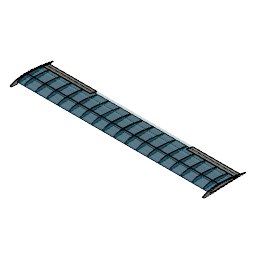
wing (Autodesk Fusion 360 design; units mm, degrees)
part number: 2026-03-18-19-06-06-757
Autodesk Fusion 360 part; units mm, degrees
(part 1 of 3)
ref_plane "WorkPlane1" through (0, 0, 0) normal (0, 0, 1) x (1, 0, 0)
sketch "Sketch2" plane through (0, 0, 0) normal (1, 0, 0) x (0, 1, 0)
  spline S0 degree 5 poles (61.12, 19.8844) (61.603, 19.9031) (62.5903, 19.9386) (64.1373, 19.9858) (66.3336, 20.0363) (69.2771, 20.0768) (72.3733, 20.092) (75.5651, 20.0792) (78.7922, 20.0358) (82.0002, 19.9602) (85.1491, 19.852) (88.221, 19.7125) (91.2143, 19.5444) (94.1405, 19.3507) (97.0192, 19.1349) (99.8745, 18.9002) (102.7305, 18.6492) (105.6069, 18.383) (108.5159, 18.1017) (111.4639, 17.8039) (114.4514, 17.4884) (117.4739, 17.1533) (120.5226, 16.7977) (123.585, 16.421) (126.6452, 16.0244) (129.6857, 15.6102) (132.6897, 15.1815) (135.6441, 14.7413) (138.5414, 14.2923) (141.3828, 13.8358) (144.1802, 13.3716) (146.96, 12.8967) (149.7596, 12.4062) (152.6192, 11.8943) (155.5748, 11.3555) (158.65, 10.7855) (161.8488, 10.1828) (165.1491, 9.5491) (168.4917, 8.8914) (171.7902, 8.2207) (174.9494, 7.5502) (177.8817, 6.8932) (180.5234, 6.2618) (182.8532, 5.6644) (184.9056, 5.1048) (186.7958, 4.5791) (188.6853, 4.0776) (190.7296, 3.5872) (193.0295, 3.0932) (195.585, 2.582) (198.2365, 2.0427) (200.7124, 1.4729) (202.699, 0.8841) (203.9033, 0.3094) (204.1194, -0.195) (203.2912, -0.5318) (201.5529, -0.6648) (199.1776, -0.6277) (196.496, -0.4891) (193.8227, -0.3307) (191.3831, -0.2214) (189.2303, -0.1908) (187.2848, -0.2357) (185.3935, -0.3335) (183.381, -0.4524) (181.1051, -0.5633) (178.5092, -0.6507) (175.6031, -0.7098) (172.4448, -0.7441) (169.123, -0.7621) (165.7378, -0.7755) (162.3835, -0.7955) (159.1292, -0.8308) (156.004, -0.8848) (153.0074, -0.9575) (150.117, -1.0461) (147.2962, -1.146) (144.5027, -1.2521) (141.6962, -1.3598) (138.8471, -1.4658) (135.9416, -1.5694) (132.9775, -1.6708) (129.9619, -1.7717) (126.9085, -1.8739) (123.8347, -1.9795) (120.7588, -2.0898) (117.6975, -2.2052) (114.6637, -2.3247) (111.6664, -2.4469) (108.7102, -2.5697) (105.7944, -2.6913) (102.9129, -2.8103) (100.0533, -2.9259) (97.1963, -3.039) (94.3176, -3.1511) (91.3932, -3.2647) (88.403, -3.3821) (85.3351, -3.5056) (82.1901, -3.6364) (78.985, -3.7745) (75.7583, -3.9183) (72.564, -4.0644) (69.462, -4.2092) (66.5097, -4.3487) (63.7533, -4.4796) (61.2187, -4.5998) (58.9035, -4.7092) (56.7672, -4.8101) (54.7458, -4.9063) (52.7684, -5.0022) (50.7726, -5.101) (48.7209, -5.2041) (46.615, -5.3099) (44.4793, -5.4149) (42.347, -5.5148) (40.2457, -5.6055) (38.181, -5.6845) (36.1282, -5.7511) (34.0511, -5.8058) (31.9176, -5.8493) (29.714, -5.8817) (27.4654, -5.9014) (25.2368, -5.9054) (23.1072, -5.8903) (21.1491, -5.8545) (19.4072, -5.799) (17.8722, -5.7297) (16.4825, -5.6547) (15.1531, -5.5769) (13.7964, -5.4879) (12.345, -5.3623) (10.7731, -5.1743) (9.1101, -4.9106) (7.4743, -4.59) (6.019, -4.2496) (4.8464, -3.9155) (3.9079, -3.575) (2.9736, -3.1567) (1.8623, -2.5675) (0.722, -1.7188) (-0.0619, -0.564) (-0.1465, 0.8714) (0.4773, 2.4376) (1.5165, 3.9094) (2.6176, 5.0911) (3.5469, 5.9078) (4.3846, 6.494) (5.3418, 7.0607) (6.5667, 7.749) (8.0285, 8.5465) (9.6168, 9.3729) (11.1943, 10.128) (12.6796, 10.7659) (14.0587, 11.2993) (15.3629, 11.7682) (16.6574, 12.2197) (18.0246, 12.6838) (19.543, 13.177) (21.2669, 13.7028) (23.2007, 14.2542) (25.2995, 14.8155) (27.4942, 15.3676) (29.7097, 15.8913) (31.8851, 16.3717) (33.9968, 16.8029) (36.0579, 17.1875) (38.0987, 17.5329) (40.1536, 17.8487) (42.246, 18.1437) (44.3706, 18.4219) (46.5002, 18.6835) (48.602, 18.9264) (50.6512, 19.1472) (52.6451, 19.3434) (54.619, 19.5144) (56.6343, 19.6612) (58.3363, 19.7608) (59.6922, 19.8261) (60.637, 19.8656) (61.12, 19.8844) knots 0 0 0 0 0 0 0.00571429 0.01142857 0.01714286 0.02285714 0.02857143 0.03428571 0.04 0.04571429 0.05142857 0.05714286 0.06285714 0.06857143 0.07428571 0.08 0.08571429 0.09142857 0.09714286 0.10285714 0.10857143 0.11428571 0.12 0.12571429 0.13142857 0.13714286 0.14285714 0.14857143 0.15428571 0.16 0.16571429 0.17142857 0.17714286 0.18285714 0.18857143 0.19428571 0.2 0.20571429 0.21142857 0.21714286 0.22285714 0.22857143 0.23428571 0.24 0.24571429 0.25142857 0.25714286 0.26285714 0.26857143 0.27428571 0.28 0.28571429 0.29142857 0.29714286 0.30285714 0.30857143 0.31428571 0.32 0.32571429 0.33142857 0.33714286 0.34285714 0.34857143 0.35428571 0.36 0.36571429 0.37142857 0.37714286 0.38285714 0.38857143 0.39428571 0.4 0.40571429 0.41142857 0.41714286 0.42285714 0.42857143 0.43428571 0.44 0.44571429 0.45142857 0.45714286 0.46285714 0.46857143 0.47428571 0.48 0.48571429 0.49142857 0.49714286 0.50285714 0.50857143 0.51428571 0.52 0.52571429 0.53142857 0.53714286 0.54285714 0.54857143 0.55428571 0.56 0.56571429 0.57142857 0.57714286 0.58285714 0.58857143 0.59428571 0.6 0.60571429 0.61142857 0.61714286 0.62285714 0.62857143 0.63428571 0.64 0.64571429 0.65142857 0.65714286 0.66285714 0.66857143 0.67428571 0.68 0.68571429 0.69142857 0.69714286 0.70285714 0.70857143 0.71428571 0.72 0.72571429 0.73142857 0.73714286 0.74285714 0.74857143 0.75428571 0.76 0.76571429 0.77142857 0.77714286 0.78285714 0.78857143 0.79428571 0.8 0.80571429 0.81142857 0.81714286 0.82285714 0.82857143 0.83428571 0.84 0.84571429 0.85142857 0.85714286 0.86285714 0.86857143 0.87428571 0.88 0.88571429 0.89142857 0.89714286 0.90285714 0.90857143 0.91428571 0.92 0.92571429 0.93142857 0.93714286 0.94285714 0.94857143 0.95428571 0.96 0.96571429 0.97142857 0.97714286 0.98285714 0.98857143 0.99428571 1 1 1 1 1 1
  line L0 (0, 0) -> (203.9051, -0.0198) construction
  point P0 (203.7334, 0.2649)
  point P1 (193.5467, 2.9949)
  point P2 (183.3601, 5.5212)
  point P3 (162.9867, 9.9626)
  point P4 (142.6134, 13.6298)
  point P5 (122.24, 16.5839)
  point P6 (101.8667, 18.7231)
  point P7 (81.4934, 19.9659)
  point P8 (61.12, 19.8844)
  point P9 (50.9334, 19.1713)
  point P10 (40.7467, 17.9285)
  point P11 (30.56, 16.0746)
  point P12 (20.3733, 13.426)
  point P13 (15.28, 11.735)
  point P14 (10.1867, 9.6366)
  point P15 (5.0933, 6.9066)
  point P16 (2.5467, 4.9711)
  point P17 (2.5467, -2.9134)
  point P18 (5.0933, -3.9728)
  point P19 (10.1867, -5.073)
  point P20 (15.28, -5.5823)
  point P21 (20.3733, -5.8268)
  point P22 (30.56, -5.8675)
  point P23 (40.7467, -5.5823)
  point P24 (50.9334, -5.0933)
  point P25 (61.12, -4.6044)
  point P26 (81.4934, -3.6672)
  point P27 (101.8667, -2.8523)
  point P28 (122.24, -2.0373)
  point P29 (142.6134, -1.3243)
  point P30 (162.9867, -0.7946)
  point P31 (183.3601, -0.4482)
  point P32 (193.5467, -0.326)
  point P33 (203.7334, -0.2649)
  point P34 (81.4934, 19.9659)
  point P35 (101.8667, 18.7231)
  point P36 (122.24, 16.5839)
  point P37 (142.6134, 13.6298)
  point P38 (162.9867, 9.9626)
  point P39 (183.3601, 5.5212)
  point P40 (193.5467, 2.9949)
  point P41 (203.7334, 0.2649)
  point P42 (203.7334, -0.2649)
  point P43 (193.5467, -0.326)
  point P44 (183.3601, -0.4482)
  point P45 (162.9867, -0.7946)
  point P46 (142.6134, -1.3243)
  point P47 (122.24, -2.0373)
  point P48 (101.8667, -2.8523)
  point P49 (81.4934, -3.6672)
  point P50 (61.12, -4.6044)
  point P51 (50.9334, -5.0933)
  point P52 (40.7467, -5.5823)
  point P53 (30.56, -5.8675)
  point P54 (20.3733, -5.8268)
  point P55 (15.28, -5.5823)
  point P56 (10.1867, -5.073)
  point P57 (5.0933, -3.9728)
  point P58 (2.5467, -2.9134)
  point P59 (2.5467, 4.9711)
  point P60 (5.0933, 6.9066)
  point P61 (10.1867, 9.6366)
  point P62 (15.28, 11.735)
  point P63 (20.3733, 13.426)
  point P64 (30.56, 16.0746)
  point P65 (40.7467, 17.9285)
  point P66 (50.9334, 19.1713)
  constraint coincident P8 S0.start
  constraint coincident P34 P7
  constraint coincident P35 P6
  constraint coincident P36 P5
  constraint coincident P37 P4
  constraint coincident P38 P3
  constraint coincident P39 P2
  constraint coincident P40 P1
  constraint coincident P41 P0
  constraint coincident P42 P33
  constraint coincident P43 P32
  constraint coincident P44 P31
  constraint coincident P45 P30
  constraint coincident P46 P29
  constraint coincident P47 P28
  constraint coincident P48 P27
  constraint coincident P49 P26
  constraint coincident P50 P25
  constraint coincident P51 P24
  constraint coincident P52 P23
  constraint coincident P53 P22
  constraint coincident P54 P21
  constraint coincident P55 P20
  constraint coincident P56 P19
  constraint coincident P57 P18
  constraint coincident P58 P17
  constraint coincident L0.start origin
  constraint coincident P59 P16
  constraint coincident P60 P15
  constraint coincident P61 P14
  constraint coincident P62 P13
  constraint coincident P63 P12
  constraint coincident P64 P11
  constraint coincident P65 P10
  constraint coincident P66 P9
  constraint coincident S0 L0.end
sketch "Sketch3" plane through (0, 0, 0) normal (0, 0, 1) x (1, 0, 0)
  line L0 (0, 0) -> (0, 200)
  line L1 (299, 155) -> (299, 200)
  line L2 (301, 200) -> (301, 155)
  line L3 (301, 155) -> (599, 155)
  line L4 (599, 155) -> (599, 200)
  line L5 (599, 200) -> (301, 200)
  line L6 (-599, 155) -> (-599, 200)
  line L7 (-301, 200) -> (-301, 155)
  line L8 (-599, 200) -> (-301, 200)
  line L9 (-299, 155) -> (-299, 200)
  line L10 (-301, 155) -> (-599, 155)
  dimension "d9" = 298
  dimension "d10" = 301
  constraint coincident L0.start origin
  constraint vertical L0
  constraint horizontal L0.end L1.end
  constraint perpendicular L2 L3
  constraint perpendicular L3 L4
  constraint perpendicular L2 L5
  constraint symmetric L0 L1.start L9.start
  constraint symmetric L0 L1.end L9.end
  constraint symmetric L0 L2.start L7.start
  constraint symmetric L0 L2.end L7.end
  constraint symmetric L0 L3.end L6.start
  constraint symmetric L0 L4.end L6.end
  measures "d9" distance of L2 L4
  measures "d10" distance of L0 L2
ref_plane "WorkPlane3" through (600, 0, 0) normal (1, 0, 0) x (0, 1, 0)
sketch "Sketch4" plane through (600, 0, 0) normal (1, 0, 0) x (0, 1, 0)
  spline S0 degree 5 poles (61.12, 19.8844) (60.637, 19.8656) (59.6922, 19.8261) (58.3363, 19.7608) (56.6343, 19.6612) (54.619, 19.5144) (52.6451, 19.3434) (50.6512, 19.1472) (48.602, 18.9264) (46.5002, 18.6835) (44.3706, 18.4219) (42.246, 18.1437) (40.1536, 17.8487) (38.0987, 17.5329) (36.0579, 17.1875) (33.9968, 16.8029) (31.8851, 16.3717) (29.7097, 15.8913) (27.4942, 15.3676) (25.2995, 14.8155) (23.2007, 14.2542) (21.2669, 13.7028) (19.543, 13.177) (18.0246, 12.6838) (16.6574, 12.2197) (15.3629, 11.7682) (14.0587, 11.2993) (12.6796, 10.7659) (11.1943, 10.128) (9.6168, 9.3729) (8.0285, 8.5465) (6.5667, 7.749) (5.3418, 7.0607) (4.3846, 6.494) (3.5469, 5.9078) (2.6176, 5.0911) (1.5165, 3.9094) (0.4773, 2.4376) (-0.1465, 0.8714) (-0.0619, -0.564) (0.722, -1.7188) (1.8623, -2.5675) (2.9736, -3.1567) (3.9079, -3.575) (4.8464, -3.9155) (6.019, -4.2496) (7.4743, -4.59) (9.1101, -4.9106) (10.7731, -5.1743) (12.345, -5.3623) (13.7964, -5.4879) (15.1531, -5.5769) (16.4825, -5.6547) (17.8722, -5.7297) (19.4072, -5.799) (21.1491, -5.8545) (23.1072, -5.8903) (25.2368, -5.9054) (27.4654, -5.9014) (29.714, -5.8817) (31.9176, -5.8493) (34.0511, -5.8058) (36.1282, -5.7511) (38.181, -5.6845) (40.2457, -5.6055) (42.347, -5.5148) (44.4793, -5.4149) (46.615, -5.3099) (48.7209, -5.2041) (50.7726, -5.101) (52.7684, -5.0022) (54.7458, -4.9063) (56.7672, -4.8101) (58.9035, -4.7092) (61.2187, -4.5998) (63.7533, -4.4796) (66.5097, -4.3487) (69.462, -4.2092) (72.564, -4.0644) (75.7583, -3.9183) (78.985, -3.7745) (82.1901, -3.6364) (85.3351, -3.5056) (88.403, -3.3821) (91.3932, -3.2647) (94.3176, -3.1511) (97.1963, -3.039) (100.0533, -2.9259) (102.9129, -2.8103) (105.7944, -2.6913) (108.7102, -2.5697) (111.6664, -2.4469) (114.6637, -2.3247) (117.6975, -2.2052) (120.7588, -2.0898) (123.8347, -1.9795) (126.9085, -1.8739) (129.9619, -1.7717) (132.9775, -1.6708) (135.9416, -1.5694) (138.8471, -1.4658) (141.6962, -1.3598) (144.5027, -1.2521) (147.2962, -1.146) (150.117, -1.0461) (153.0074, -0.9575) (156.004, -0.8848) (159.1292, -0.8308) (162.3835, -0.7955) (165.7378, -0.7755) (169.123, -0.7621) (172.4448, -0.7441) (175.6031, -0.7098) (178.5092, -0.6507) (181.1051, -0.5633) (183.381, -0.4524) (185.3935, -0.3335) (187.2848, -0.2357) (189.2303, -0.1908) (191.3831, -0.2214) (193.8227, -0.3307) (196.496, -0.4891) (199.1776, -0.6277) (201.5529, -0.6648) (203.2912, -0.5318) (204.1194, -0.195) (203.9033, 0.3094) (202.699, 0.8841) (200.7124, 1.4729) (198.2365, 2.0427) (195.585, 2.582) (193.0295, 3.0932) (190.7296, 3.5872) (188.6853, 4.0776) (186.7958, 4.5791) (184.9056, 5.1048) (182.8532, 5.6644) (180.5234, 6.2618) (177.8817, 6.8932) (174.9494, 7.5502) (171.7902, 8.2207) (168.4917, 8.8914) (165.1491, 9.5491) (161.8488, 10.1828) (158.65, 10.7855) (155.5748, 11.3555) (152.6192, 11.8943) (149.7596, 12.4062) (146.96, 12.8967) (144.1802, 13.3716) (141.3828, 13.8358) (138.5414, 14.2923) (135.6441, 14.7413) (132.6897, 15.1815) (129.6857, 15.6102) (126.6452, 16.0244) (123.585, 16.421) (120.5226, 16.7977) (117.4739, 17.1533) (114.4514, 17.4884) (111.4639, 17.8039) (108.5159, 18.1017) (105.6069, 18.383) (102.7305, 18.6492) (99.8745, 18.9002) (97.0192, 19.1349) (94.1405, 19.3507) (91.2143, 19.5444) (88.221, 19.7125) (85.1491, 19.852) (82.0002, 19.9602) (78.7922, 20.0358) (75.5651, 20.0792) (72.3733, 20.092) (69.2771, 20.0768) (66.3336, 20.0363) (64.1373, 19.9858) (62.5903, 19.9386) (61.603, 19.9031) (61.12, 19.8844) knots -1 -1 -1 -1 -1 -1 -0.99428571 -0.98857143 -0.98285714 -0.97714286 -0.97142857 -0.96571429 -0.96 -0.95428571 -0.94857143 -0.94285714 -0.93714286 -0.93142857 -0.92571429 -0.92 -0.91428571 -0.90857143 -0.90285714 -0.89714286 -0.89142857 -0.88571429 -0.88 -0.87428571 -0.86857143 -0.86285714 -0.85714286 -0.85142857 -0.84571429 -0.84 -0.83428571 -0.82857143 -0.82285714 -0.81714286 -0.81142857 -0.80571429 -0.8 -0.79428571 -0.78857143 -0.78285714 -0.77714286 -0.77142857 -0.76571429 -0.76 -0.75428571 -0.74857143 -0.74285714 -0.73714286 -0.73142857 -0.72571429 -0.72 -0.71428571 -0.70857143 -0.70285714 -0.69714286 -0.69142857 -0.68571429 -0.68 -0.67428571 -0.66857143 -0.66285714 -0.65714286 -0.65142857 -0.64571429 -0.64 -0.63428571 -0.62857143 -0.62285714 -0.61714286 -0.61142857 -0.60571429 -0.6 -0.59428571 -0.58857143 -0.58285714 -0.57714286 -0.57142857 -0.56571429 -0.56 -0.55428571 -0.54857143 -0.54285714 -0.53714286 -0.53142857 -0.52571429 -0.52 -0.51428571 -0.50857143 -0.50285714 -0.49714286 -0.49142857 -0.48571429 -0.48 -0.47428571 -0.46857143 -0.46285714 -0.45714286 -0.45142857 -0.44571429 -0.44 -0.43428571 -0.42857143 -0.42285714 -0.41714286 -0.41142857 -0.40571429 -0.4 -0.39428571 -0.38857143 -0.38285714 -0.37714286 -0.37142857 -0.36571429 -0.36 -0.35428571 -0.34857143 -0.34285714 -0.33714286 -0.33142857 -0.32571429 -0.32 -0.31428571 -0.30857143 -0.30285714 -0.29714286 -0.29142857 -0.28571429 -0.28 -0.27428571 -0.26857143 -0.26285714 -0.25714286 -0.25142857 -0.24571429 -0.24 -0.23428571 -0.22857143 -0.22285714 -0.21714286 -0.21142857 -0.20571429 -0.2 -0.19428571 -0.18857143 -0.18285714 -0.17714286 -0.17142857 -0.16571429 -0.16 -0.15428571 -0.14857143 -0.14285714 -0.13714286 -0.13142857 -0.12571429 -0.12 -0.11428571 -0.10857143 -0.10285714 -0.09714286 -0.09142857 -0.08571429 -0.08 -0.07428571 -0.06857143 -0.06285714 -0.05714286 -0.05142857 -0.04571429 -0.04 -0.03428571 -0.02857143 -0.02285714 -0.01714286 -0.01142857 -0.00571429 0 0 0 0 0 0
  spline S1 degree 3 poles (61.2364, 16.8866) (57.6324, 16.7467) (54.837, 16.5421) (51.8513, 16.2482) (49.2932, 15.9964) (46.5535, 15.6792) (43.8366, 15.324) (41.401, 15.0055) (39.0596, 14.6628) (36.7294, 14.2509) (34.6015, 13.8747) (32.4156, 13.4278) (30.1291, 12.901) (27.6916, 12.3395) (25.1848, 11.6956) (23.0631, 11.091) (21.2216, 10.5662) (19.7064, 10.0816) (18.3739, 9.632) (16.6918, 9.0644) (15.2258, 8.5644) (13.5524, 7.8653) (12.4462, 7.4031) (11.2189, 6.8194) (9.9999, 6.1844) (8.9215, 5.6226) (7.8857, 5.0512) (7.1019, 4.6035) (6.4838, 4.2504) (6.0525, 3.9896) (5.6921, 3.7303) (5.3517, 3.4854) (5.0032, 3.1949) (4.5699, 2.7504) (4.1116, 2.2804) (3.595, 1.6449) (3.2914, 1.117) (3.1087, 0.7992) (3.0156, 0.5398) (2.9897, 0.42) knots -1 -1 -1 -1 -0.97404 -0.97404 -0.97404 -0.951798 -0.951798 -0.951798 -0.931858 -0.931858 -0.931858 -0.913649 -0.913649 -0.913649 -0.894237 -0.894237 -0.894237 -0.877389 -0.877389 -0.877389 -0.856122 -0.856122 -0.856122 -0.842064 -0.842064 -0.842064 -0.829628 -0.829628 -0.829628 -0.819821 -0.819821 -0.819821 -0.810556 -0.810556 -0.810556 -0.800757 -0.800757 -0.800757 -0.79486 -0.79486 -0.79486 -0.79486
  spline S2 degree 3 poles (2.9897, 0.42) (3.0543, 0.3464) (3.1943, 0.219) (3.3872, 0.0837) (3.7574, -0.176) (4.273, -0.4422) (4.7124, -0.6375) (5.2684, -0.8846) (5.7621, -1.0583) (6.571, -1.2759) (7.6681, -1.5709) (9.285, -1.9057) (10.7983, -2.1313) (12.3486, -2.3624) (13.7433, -2.4772) (15.0921, -2.5644) (16.7453, -2.6714) (18.3654, -2.7647) (20.5139, -2.8297) (22.493, -2.8895) (24.9582, -2.9109) (27.506, -2.8972) (29.7799, -2.8851) (32.0483, -2.8498) (34.1902, -2.7985) (36.8126, -2.7357) (39.3288, -2.6442) (41.9726, -2.5266) (44.569, -2.411) (47.2437, -2.2742) (49.7746, -2.1475) (52.1544, -2.0283) (54.3796, -1.9201) (56.8136, -1.8047) (59.0608, -1.6981) (61.5509, -1.5807) (64.4566, -1.4428) (69.9758, -1.181) (76.92, -0.8547) (83.3434, -0.5864) (87.9529, -0.3939) (92.2873, -0.2286) (96.4895, -0.064) (101.2103, 0.121) (105.8624, 0.3155) (110.7376, 0.5168) (116.1156, 0.7389) (121.7528, 0.9526) (127.3, 1.1404) (131.5605, 1.2846) (135.7191, 1.4217) (139.6944, 1.5684) (145.3748, 1.778) (150.7153, 2.0131) (156.9225, 2.1285) (160.1948, 2.1893) (163.72, 2.2137) (167.2511, 2.2303) (171.3919, 2.2497) (175.4512, 2.2724) (178.7296, 2.3656) (180.2835, 2.4098) (181.6615, 2.4681) (182.9209, 2.533) knots -0.783322 -0.783322 -0.783322 -0.783322 -0.778142 -0.778142 -0.778142 -0.768195 -0.768195 -0.768195 -0.755608 -0.755608 -0.755608 -0.738537 -0.738537 -0.738537 -0.721048 -0.721048 -0.721048 -0.699613 -0.699613 -0.699613 -0.679868 -0.679868 -0.679868 -0.662246 -0.662246 -0.662246 -0.640672 -0.640672 -0.640672 -0.619485 -0.619485 -0.619485 -0.599563 -0.599563 -0.599563 -0.58117 -0.58117 -0.58117 -0.546233 -0.546233 -0.546233 -0.521162 -0.521162 -0.521162 -0.492997 -0.492997 -0.492997 -0.461927 -0.461927 -0.461927 -0.438064 -0.438064 -0.438064 -0.403967 -0.403967 -0.403967 -0.385991 -0.385991 -0.385991 -0.364912 -0.364912 -0.364912 -0.354921 -0.354921 -0.354921 -0.354921
  spline S3 degree 3 poles (182.9209, 2.533) (181.8753, 2.8143) (180.7522, 3.1063) (179.5028, 3.4129) (176.8181, 4.0717) (173.5306, 4.7965) (170.0047, 5.5188) (166.4626, 6.2444) (162.7518, 6.9595) (159.2882, 7.6111) (155.1437, 8.3909) (151.3487, 9.0818) (147.6957, 9.7206) (143.9527, 10.3752) (140.28, 10.987) (136.4155, 11.5838) (130.3032, 12.5277) (123.7504, 13.4125) (117.3527, 14.1433) (112.3122, 14.7191) (107.4083, 15.2105) (102.6424, 15.6416) (98.0281, 16.059) (93.5117, 16.421) (88.6866, 16.6762) (85.0421, 16.869) (81.1898, 16.9968) (77.299, 17.0516) (73.1641, 17.1099) (69.0475, 17.0885) (65.4867, 17.0124) (63.97, 16.9799) (62.5517, 16.9377) (61.2364, 16.8866) knots -0.236727 -0.236727 -0.236727 -0.236727 -0.22805 -0.22805 -0.22805 -0.209405 -0.209405 -0.209405 -0.190675 -0.190675 -0.190675 -0.168261 -0.168261 -0.168261 -0.145296 -0.145296 -0.145296 -0.108972 -0.108972 -0.108972 -0.080353 -0.080353 -0.080353 -0.052644 -0.052644 -0.052644 -0.031716 -0.031716 -0.031716 -0.009474 -0.009474 -0.009474 0 0 0 0
  dimension "d12" = -3
extrude "Extrude2" add sketch "Sketch4" against normal blind 1200 makes body 1
sketch "Sketch5" plane through (600, 0, 0) normal (1, 0, 0) x (0, 1, 0)
  spline S0 degree 5 poles (61.12, 19.8844) (60.637, 19.8656) (59.6922, 19.8261) (58.3363, 19.7608) (56.6343, 19.6612) (54.619, 19.5144) (52.6451, 19.3434) (50.6512, 19.1472) (48.602, 18.9264) (46.5002, 18.6835) (44.3706, 18.4219) (42.246, 18.1437) (40.1536, 17.8487) (38.0987, 17.5329) (36.0579, 17.1875) (33.9968, 16.8029) (31.8851, 16.3717) (29.7097, 15.8913) (27.4942, 15.3676) (25.2995, 14.8155) (23.2007, 14.2542) (21.2669, 13.7028) (19.543, 13.177) (18.0246, 12.6838) (16.6574, 12.2197) (15.3629, 11.7682) (14.0587, 11.2993) (12.6796, 10.7659) (11.1943, 10.128) (9.6168, 9.3729) (8.0285, 8.5465) (6.5667, 7.749) (5.3418, 7.0607) (4.3846, 6.494) (3.5469, 5.9078) (2.6176, 5.0911) (1.5165, 3.9094) (0.4773, 2.4376) (-0.1465, 0.8714) (-0.0619, -0.564) (0.722, -1.7188) (1.8623, -2.5675) (2.9736, -3.1567) (3.9079, -3.575) (4.8464, -3.9155) (6.019, -4.2496) (7.4743, -4.59) (9.1101, -4.9106) (10.7731, -5.1743) (12.345, -5.3623) (13.7964, -5.4879) (15.1531, -5.5769) (16.4825, -5.6547) (17.8722, -5.7297) (19.4072, -5.799) (21.1491, -5.8545) (23.1072, -5.8903) (25.2368, -5.9054) (27.4654, -5.9014) (29.714, -5.8817) (31.9176, -5.8493) (34.0511, -5.8058) (36.1282, -5.7511) (38.181, -5.6845) (40.2457, -5.6055) (42.347, -5.5148) (44.4793, -5.4149) (46.615, -5.3099) (48.7209, -5.2041) (50.7726, -5.101) (52.7684, -5.0022) (54.7458, -4.9063) (56.7672, -4.8101) (58.9035, -4.7092) (61.2187, -4.5998) (63.7533, -4.4796) (66.5097, -4.3487) (69.462, -4.2092) (72.564, -4.0644) (75.7583, -3.9183) (78.985, -3.7745) (82.1901, -3.6364) (85.3351, -3.5056) (88.403, -3.3821) (91.3932, -3.2647) (94.3176, -3.1511) (97.1963, -3.039) (100.0533, -2.9259) (102.9129, -2.8103) (105.7944, -2.6913) (108.7102, -2.5697) (111.6664, -2.4469) (114.6637, -2.3247) (117.6975, -2.2052) (120.7588, -2.0898) (123.8347, -1.9795) (126.9085, -1.8739) (129.9619, -1.7717) (132.9775, -1.6708) (135.9416, -1.5694) (138.8471, -1.4658) (141.6962, -1.3598) (144.5027, -1.2521) (147.2962, -1.146) (150.117, -1.0461) (153.0074, -0.9575) (156.004, -0.8848) (159.1292, -0.8308) (162.3835, -0.7955) (165.7378, -0.7755) (169.123, -0.7621) (172.4448, -0.7441) (175.6031, -0.7098) (178.5092, -0.6507) (181.1051, -0.5633) (183.381, -0.4524) (185.3935, -0.3335) (187.2848, -0.2357) (189.2303, -0.1908) (191.3831, -0.2214) (193.8227, -0.3307) (196.496, -0.4891) (199.1776, -0.6277) (201.5529, -0.6648) (203.2912, -0.5318) (204.1194, -0.195) (203.9033, 0.3094) (202.699, 0.8841) (200.7124, 1.4729) (198.2365, 2.0427) (195.585, 2.582) (193.0295, 3.0932) (190.7296, 3.5872) (188.6853, 4.0776) (186.7958, 4.5791) (184.9056, 5.1048) (182.8532, 5.6644) (180.5234, 6.2618) (177.8817, 6.8932) (174.9494, 7.5502) (171.7902, 8.2207) (168.4917, 8.8914) (165.1491, 9.5491) (161.8488, 10.1828) (158.65, 10.7855) (155.5748, 11.3555) (152.6192, 11.8943) (149.7596, 12.4062) (146.96, 12.8967) (144.1802, 13.3716) (141.3828, 13.8358) (138.5414, 14.2923) (135.6441, 14.7413) (132.6897, 15.1815) (129.6857, 15.6102) (126.6452, 16.0244) (123.585, 16.421) (120.5226, 16.7977) (117.4739, 17.1533) (114.4514, 17.4884) (111.4639, 17.8039) (108.5159, 18.1017) (105.6069, 18.383) (102.7305, 18.6492) (99.8745, 18.9002) (97.0192, 19.1349) (94.1405, 19.3507) (91.2143, 19.5444) (88.221, 19.7125) (85.1491, 19.852) (82.0002, 19.9602) (78.7922, 20.0358) (75.5651, 20.0792) (72.3733, 20.092) (69.2771, 20.0768) (66.3336, 20.0363) (64.1373, 19.9858) (62.5903, 19.9386) (61.603, 19.9031) (61.12, 19.8844) knots -1 -1 -1 -1 -1 -1 -0.99428571 -0.98857143 -0.98285714 -0.97714286 -0.97142857 -0.96571429 -0.96 -0.95428571 -0.94857143 -0.94285714 -0.93714286 -0.93142857 -0.92571429 -0.92 -0.91428571 -0.90857143 -0.90285714 -0.89714286 -0.89142857 -0.88571429 -0.88 -0.87428571 -0.86857143 -0.86285714 -0.85714286 -0.85142857 -0.84571429 -0.84 -0.83428571 -0.82857143 -0.82285714 -0.81714286 -0.81142857 -0.80571429 -0.8 -0.79428571 -0.78857143 -0.78285714 -0.77714286 -0.77142857 -0.76571429 -0.76 -0.75428571 -0.74857143 -0.74285714 -0.73714286 -0.73142857 -0.72571429 -0.72 -0.71428571 -0.70857143 -0.70285714 -0.69714286 -0.69142857 -0.68571429 -0.68 -0.67428571 -0.66857143 -0.66285714 -0.65714286 -0.65142857 -0.64571429 -0.64 -0.63428571 -0.62857143 -0.62285714 -0.61714286 -0.61142857 -0.60571429 -0.6 -0.59428571 -0.58857143 -0.58285714 -0.57714286 -0.57142857 -0.56571429 -0.56 -0.55428571 -0.54857143 -0.54285714 -0.53714286 -0.53142857 -0.52571429 -0.52 -0.51428571 -0.50857143 -0.50285714 -0.49714286 -0.49142857 -0.48571429 -0.48 -0.47428571 -0.46857143 -0.46285714 -0.45714286 -0.45142857 -0.44571429 -0.44 -0.43428571 -0.42857143 -0.42285714 -0.41714286 -0.41142857 -0.40571429 -0.4 -0.39428571 -0.38857143 -0.38285714 -0.37714286 -0.37142857 -0.36571429 -0.36 -0.35428571 -0.34857143 -0.34285714 -0.33714286 -0.33142857 -0.32571429 -0.32 -0.31428571 -0.30857143 -0.30285714 -0.29714286 -0.29142857 -0.28571429 -0.28 -0.27428571 -0.26857143 -0.26285714 -0.25714286 -0.25142857 -0.24571429 -0.24 -0.23428571 -0.22857143 -0.22285714 -0.21714286 -0.21142857 -0.20571429 -0.2 -0.19428571 -0.18857143 -0.18285714 -0.17714286 -0.17142857 -0.16571429 -0.16 -0.15428571 -0.14857143 -0.14285714 -0.13714286 -0.13142857 -0.12571429 -0.12 -0.11428571 -0.10857143 -0.10285714 -0.09714286 -0.09142857 -0.08571429 -0.08 -0.07428571 -0.06857143 -0.06285714 -0.05714286 -0.05142857 -0.04571429 -0.04 -0.03428571 -0.02857143 -0.02285714 -0.01714286 -0.01142857 -0.00571429 0 0 0 0 0 0
sketch "Sketch6" plane through (600, 0, 0) normal (1, 0, 0) x (0, 1, 0)
  spline S0 degree 5 poles (61.12, 19.8844) (60.637, 19.8656) (59.6922, 19.8261) (58.3363, 19.7608) (56.6343, 19.6612) (54.619, 19.5144) (52.6451, 19.3434) (50.6512, 19.1472) (48.602, 18.9264) (46.5002, 18.6835) (44.3706, 18.4219) (42.246, 18.1437) (40.1536, 17.8487) (38.0987, 17.5329) (36.0579, 17.1875) (33.9968, 16.8029) (31.8851, 16.3717) (29.7097, 15.8913) (27.4942, 15.3676) (25.2995, 14.8155) (23.2007, 14.2542) (21.2669, 13.7028) (19.543, 13.177) (18.0246, 12.6838) (16.6574, 12.2197) (15.3629, 11.7682) (14.0587, 11.2993) (12.6796, 10.7659) (11.1943, 10.128) (9.6168, 9.3729) (8.0285, 8.5465) (6.5667, 7.749) (5.3418, 7.0607) (4.3846, 6.494) (3.5469, 5.9078) (2.6176, 5.0911) (1.5165, 3.9094) (0.4773, 2.4376) (-0.1465, 0.8714) (-0.0619, -0.564) (0.722, -1.7188) (1.8623, -2.5675) (2.9736, -3.1567) (3.9079, -3.575) (4.8464, -3.9155) (6.019, -4.2496) (7.4743, -4.59) (9.1101, -4.9106) (10.7731, -5.1743) (12.345, -5.3623) (13.7964, -5.4879) (15.1531, -5.5769) (16.4825, -5.6547) (17.8722, -5.7297) (19.4072, -5.799) (21.1491, -5.8545) (23.1072, -5.8903) (25.2368, -5.9054) (27.4654, -5.9014) (29.714, -5.8817) (31.9176, -5.8493) (34.0511, -5.8058) (36.1282, -5.7511) (38.181, -5.6845) (40.2457, -5.6055) (42.347, -5.5148) (44.4793, -5.4149) (46.615, -5.3099) (48.7209, -5.2041) (50.7726, -5.101) (52.7684, -5.0022) (54.7458, -4.9063) (56.7672, -4.8101) (58.9035, -4.7092) (61.2187, -4.5998) (63.7533, -4.4796) (66.5097, -4.3487) (69.462, -4.2092) (72.564, -4.0644) (75.7583, -3.9183) (78.985, -3.7745) (82.1901, -3.6364) (85.3351, -3.5056) (88.403, -3.3821) (91.3932, -3.2647) (94.3176, -3.1511) (97.1963, -3.039) (100.0533, -2.9259) (102.9129, -2.8103) (105.7944, -2.6913) (108.7102, -2.5697) (111.6664, -2.4469) (114.6637, -2.3247) (117.6975, -2.2052) (120.7588, -2.0898) (123.8347, -1.9795) (126.9085, -1.8739) (129.9619, -1.7717) (132.9775, -1.6708) (135.9416, -1.5694) (138.8471, -1.4658) (141.6962, -1.3598) (144.5027, -1.2521) (147.2962, -1.146) (150.117, -1.0461) (153.0074, -0.9575) (156.004, -0.8848) (159.1292, -0.8308) (162.3835, -0.7955) (165.7378, -0.7755) (169.123, -0.7621) (172.4448, -0.7441) (175.6031, -0.7098) (178.5092, -0.6507) (181.1051, -0.5633) (183.381, -0.4524) (185.3935, -0.3335) (187.2848, -0.2357) (189.2303, -0.1908) (191.3831, -0.2214) (193.8227, -0.3307) (196.496, -0.4891) (199.1776, -0.6277) (201.5529, -0.6648) (203.2912, -0.5318) (204.1194, -0.195) (203.9033, 0.3094) (202.699, 0.8841) (200.7124, 1.4729) (198.2365, 2.0427) (195.585, 2.582) (193.0295, 3.0932) (190.7296, 3.5872) (188.6853, 4.0776) (186.7958, 4.5791) (184.9056, 5.1048) (182.8532, 5.6644) (180.5234, 6.2618) (177.8817, 6.8932) (174.9494, 7.5502) (171.7902, 8.2207) (168.4917, 8.8914) (165.1491, 9.5491) (161.8488, 10.1828) (158.65, 10.7855) (155.5748, 11.3555) (152.6192, 11.8943) (149.7596, 12.4062) (146.96, 12.8967) (144.1802, 13.3716) (141.3828, 13.8358) (138.5414, 14.2923) (135.6441, 14.7413) (132.6897, 15.1815) (129.6857, 15.6102) (126.6452, 16.0244) (123.585, 16.421) (120.5226, 16.7977) (117.4739, 17.1533) (114.4514, 17.4884) (111.4639, 17.8039) (108.5159, 18.1017) (105.6069, 18.383) (102.7305, 18.6492) (99.8745, 18.9002) (97.0192, 19.1349) (94.1405, 19.3507) (91.2143, 19.5444) (88.221, 19.7125) (85.1491, 19.852) (82.0002, 19.9602) (78.7922, 20.0358) (75.5651, 20.0792) (72.3733, 20.092) (69.2771, 20.0768) (66.3336, 20.0363) (64.1373, 19.9858) (62.5903, 19.9386) (61.603, 19.9031) (61.12, 19.8844) knots -1 -1 -1 -1 -1 -1 -0.99428571 -0.98857143 -0.98285714 -0.97714286 -0.97142857 -0.96571429 -0.96 -0.95428571 -0.94857143 -0.94285714 -0.93714286 -0.93142857 -0.92571429 -0.92 -0.91428571 -0.90857143 -0.90285714 -0.89714286 -0.89142857 -0.88571429 -0.88 -0.87428571 -0.86857143 -0.86285714 -0.85714286 -0.85142857 -0.84571429 -0.84 -0.83428571 -0.82857143 -0.82285714 -0.81714286 -0.81142857 -0.80571429 -0.8 -0.79428571 -0.78857143 -0.78285714 -0.77714286 -0.77142857 -0.76571429 -0.76 -0.75428571 -0.74857143 -0.74285714 -0.73714286 -0.73142857 -0.72571429 -0.72 -0.71428571 -0.70857143 -0.70285714 -0.69714286 -0.69142857 -0.68571429 -0.68 -0.67428571 -0.66857143 -0.66285714 -0.65714286 -0.65142857 -0.64571429 -0.64 -0.63428571 -0.62857143 -0.62285714 -0.61714286 -0.61142857 -0.60571429 -0.6 -0.59428571 -0.58857143 -0.58285714 -0.57714286 -0.57142857 -0.56571429 -0.56 -0.55428571 -0.54857143 -0.54285714 -0.53714286 -0.53142857 -0.52571429 -0.52 -0.51428571 -0.50857143 -0.50285714 -0.49714286 -0.49142857 -0.48571429 -0.48 -0.47428571 -0.46857143 -0.46285714 -0.45714286 -0.45142857 -0.44571429 -0.44 -0.43428571 -0.42857143 -0.42285714 -0.41714286 -0.41142857 -0.40571429 -0.4 -0.39428571 -0.38857143 -0.38285714 -0.37714286 -0.37142857 -0.36571429 -0.36 -0.35428571 -0.34857143 -0.34285714 -0.33714286 -0.33142857 -0.32571429 -0.32 -0.31428571 -0.30857143 -0.30285714 -0.29714286 -0.29142857 -0.28571429 -0.28 -0.27428571 -0.26857143 -0.26285714 -0.25714286 -0.25142857 -0.24571429 -0.24 -0.23428571 -0.22857143 -0.22285714 -0.21714286 -0.21142857 -0.20571429 -0.2 -0.19428571 -0.18857143 -0.18285714 -0.17714286 -0.17142857 -0.16571429 -0.16 -0.15428571 -0.14857143 -0.14285714 -0.13714286 -0.13142857 -0.12571429 -0.12 -0.11428571 -0.10857143 -0.10285714 -0.09714286 -0.09142857 -0.08571429 -0.08 -0.07428571 -0.06857143 -0.06285714 -0.05714286 -0.05142857 -0.04571429 -0.04 -0.03428571 -0.02857143 -0.02285714 -0.01714286 -0.01142857 -0.00571429 0 0 0 0 0 0
sketch "Sketch7" plane through (600, 0, 0) normal (1, 0, 0) x (0, 1, 0)
  spline S0 degree 5 poles (61.12, 19.8844) (60.637, 19.8656) (59.6922, 19.8261) (58.3363, 19.7608) (56.6343, 19.6612) (54.619, 19.5144) (52.6451, 19.3434) (50.6512, 19.1472) (48.602, 18.9264) (46.5002, 18.6835) (44.3706, 18.4219) (42.246, 18.1437) (40.1536, 17.8487) (38.0987, 17.5329) (36.0579, 17.1875) (33.9968, 16.8029) (31.8851, 16.3717) (29.7097, 15.8913) (27.4942, 15.3676) (25.2995, 14.8155) (23.2007, 14.2542) (21.2669, 13.7028) (19.543, 13.177) (18.0246, 12.6838) (16.6574, 12.2197) (15.3629, 11.7682) (14.0587, 11.2993) (12.6796, 10.7659) (11.1943, 10.128) (9.6168, 9.3729) (8.0285, 8.5465) (6.5667, 7.749) (5.3418, 7.0607) (4.3846, 6.494) (3.5469, 5.9078) (2.6176, 5.0911) (1.5165, 3.9094) (0.4773, 2.4376) (-0.1465, 0.8714) (-0.0619, -0.564) (0.722, -1.7188) (1.8623, -2.5675) (2.9736, -3.1567) (3.9079, -3.575) (4.8464, -3.9155) (6.019, -4.2496) (7.4743, -4.59) (9.1101, -4.9106) (10.7731, -5.1743) (12.345, -5.3623) (13.7964, -5.4879) (15.1531, -5.5769) (16.4825, -5.6547) (17.8722, -5.7297) (19.4072, -5.799) (21.1491, -5.8545) (23.1072, -5.8903) (25.2368, -5.9054) (27.4654, -5.9014) (29.714, -5.8817) (31.9176, -5.8493) (34.0511, -5.8058) (36.1282, -5.7511) (38.181, -5.6845) (40.2457, -5.6055) (42.347, -5.5148) (44.4793, -5.4149) (46.615, -5.3099) (48.7209, -5.2041) (50.7726, -5.101) (52.7684, -5.0022) (54.7458, -4.9063) (56.7672, -4.8101) (58.9035, -4.7092) (61.2187, -4.5998) (63.7533, -4.4796) (66.5097, -4.3487) (69.462, -4.2092) (72.564, -4.0644) (75.7583, -3.9183) (78.985, -3.7745) (82.1901, -3.6364) (85.3351, -3.5056) (88.403, -3.3821) (91.3932, -3.2647) (94.3176, -3.1511) (97.1963, -3.039) (100.0533, -2.9259) (102.9129, -2.8103) (105.7944, -2.6913) (108.7102, -2.5697) (111.6664, -2.4469) (114.6637, -2.3247) (117.6975, -2.2052) (120.7588, -2.0898) (123.8347, -1.9795) (126.9085, -1.8739) (129.9619, -1.7717) (132.9775, -1.6708) (135.9416, -1.5694) (138.8471, -1.4658) (141.6962, -1.3598) (144.5027, -1.2521) (147.2962, -1.146) (150.117, -1.0461) (153.0074, -0.9575) (156.004, -0.8848) (159.1292, -0.8308) (162.3835, -0.7955) (165.7378, -0.7755) (169.123, -0.7621) (172.4448, -0.7441) (175.6031, -0.7098) (178.5092, -0.6507) (181.1051, -0.5633) (183.381, -0.4524) (185.3935, -0.3335) (187.2848, -0.2357) (189.2303, -0.1908) (191.3831, -0.2214) (193.8227, -0.3307) (196.496, -0.4891) (199.1776, -0.6277) (201.5529, -0.6648) (203.2912, -0.5318) (204.1194, -0.195) (203.9033, 0.3094) (202.699, 0.8841) (200.7124, 1.4729) (198.2365, 2.0427) (195.585, 2.582) (193.0295, 3.0932) (190.7296, 3.5872) (188.6853, 4.0776) (186.7958, 4.5791) (184.9056, 5.1048) (182.8532, 5.6644) (180.5234, 6.2618) (177.8817, 6.8932) (174.9494, 7.5502) (171.7902, 8.2207) (168.4917, 8.8914) (165.1491, 9.5491) (161.8488, 10.1828) (158.65, 10.7855) (155.5748, 11.3555) (152.6192, 11.8943) (149.7596, 12.4062) (146.96, 12.8967) (144.1802, 13.3716) (141.3828, 13.8358) (138.5414, 14.2923) (135.6441, 14.7413) (132.6897, 15.1815) (129.6857, 15.6102) (126.6452, 16.0244) (123.585, 16.421) (120.5226, 16.7977) (117.4739, 17.1533) (114.4514, 17.4884) (111.4639, 17.8039) (108.5159, 18.1017) (105.6069, 18.383) (102.7305, 18.6492) (99.8745, 18.9002) (97.0192, 19.1349) (94.1405, 19.3507) (91.2143, 19.5444) (88.221, 19.7125) (85.1491, 19.852) (82.0002, 19.9602) (78.7922, 20.0358) (75.5651, 20.0792) (72.3733, 20.092) (69.2771, 20.0768) (66.3336, 20.0363) (64.1373, 19.9858) (62.5903, 19.9386) (61.603, 19.9031) (61.12, 19.8844) knots -1 -1 -1 -1 -1 -1 -0.99428571 -0.98857143 -0.98285714 -0.97714286 -0.97142857 -0.96571429 -0.96 -0.95428571 -0.94857143 -0.94285714 -0.93714286 -0.93142857 -0.92571429 -0.92 -0.91428571 -0.90857143 -0.90285714 -0.89714286 -0.89142857 -0.88571429 -0.88 -0.87428571 -0.86857143 -0.86285714 -0.85714286 -0.85142857 -0.84571429 -0.84 -0.83428571 -0.82857143 -0.82285714 -0.81714286 -0.81142857 -0.80571429 -0.8 -0.79428571 -0.78857143 -0.78285714 -0.77714286 -0.77142857 -0.76571429 -0.76 -0.75428571 -0.74857143 -0.74285714 -0.73714286 -0.73142857 -0.72571429 -0.72 -0.71428571 -0.70857143 -0.70285714 -0.69714286 -0.69142857 -0.68571429 -0.68 -0.67428571 -0.66857143 -0.66285714 -0.65714286 -0.65142857 -0.64571429 -0.64 -0.63428571 -0.62857143 -0.62285714 -0.61714286 -0.61142857 -0.60571429 -0.6 -0.59428571 -0.58857143 -0.58285714 -0.57714286 -0.57142857 -0.56571429 -0.56 -0.55428571 -0.54857143 -0.54285714 -0.53714286 -0.53142857 -0.52571429 -0.52 -0.51428571 -0.50857143 -0.50285714 -0.49714286 -0.49142857 -0.48571429 -0.48 -0.47428571 -0.46857143 -0.46285714 -0.45714286 -0.45142857 -0.44571429 -0.44 -0.43428571 -0.42857143 -0.42285714 -0.41714286 -0.41142857 -0.40571429 -0.4 -0.39428571 -0.38857143 -0.38285714 -0.37714286 -0.37142857 -0.36571429 -0.36 -0.35428571 -0.34857143 -0.34285714 -0.33714286 -0.33142857 -0.32571429 -0.32 -0.31428571 -0.30857143 -0.30285714 -0.29714286 -0.29142857 -0.28571429 -0.28 -0.27428571 -0.26857143 -0.26285714 -0.25714286 -0.25142857 -0.24571429 -0.24 -0.23428571 -0.22857143 -0.22285714 -0.21714286 -0.21142857 -0.20571429 -0.2 -0.19428571 -0.18857143 -0.18285714 -0.17714286 -0.17142857 -0.16571429 -0.16 -0.15428571 -0.14857143 -0.14285714 -0.13714286 -0.13142857 -0.12571429 -0.12 -0.11428571 -0.10857143 -0.10285714 -0.09714286 -0.09142857 -0.08571429 -0.08 -0.07428571 -0.06857143 -0.06285714 -0.05714286 -0.05142857 -0.04571429 -0.04 -0.03428571 -0.02857143 -0.02285714 -0.01714286 -0.01142857 -0.00571429 0 0 0 0 0 0
  spline S1 degree 3 poles (61.2364, 16.8866) (57.6324, 16.7467) (54.837, 16.5421) (51.8513, 16.2482) (49.2932, 15.9964) (46.5535, 15.6792) (43.8366, 15.324) (41.401, 15.0055) (39.0596, 14.6628) (36.7294, 14.2509) (34.6015, 13.8747) (32.4156, 13.4278) (30.1291, 12.901) (27.6916, 12.3395) (25.1848, 11.6956) (23.0631, 11.091) (21.2216, 10.5662) (19.7064, 10.0816) (18.3739, 9.632) (16.6918, 9.0644) (15.2258, 8.5644) (13.5524, 7.8653) (12.4462, 7.4031) (11.2189, 6.8194) (9.9999, 6.1844) (8.9215, 5.6226) (7.8857, 5.0512) (7.1019, 4.6035) (6.4838, 4.2504) (6.0525, 3.9896) (5.6921, 3.7303) (5.3517, 3.4854) (5.0032, 3.1949) (4.5699, 2.7504) (4.1116, 2.2804) (3.595, 1.6449) (3.2914, 1.117) (3.1087, 0.7992) (3.0156, 0.5398) (2.9897, 0.42) knots -1 -1 -1 -1 -0.97404 -0.97404 -0.97404 -0.951798 -0.951798 -0.951798 -0.931858 -0.931858 -0.931858 -0.913649 -0.913649 -0.913649 -0.894237 -0.894237 -0.894237 -0.877389 -0.877389 -0.877389 -0.856122 -0.856122 -0.856122 -0.842064 -0.842064 -0.842064 -0.829628 -0.829628 -0.829628 -0.819821 -0.819821 -0.819821 -0.810556 -0.810556 -0.810556 -0.800757 -0.800757 -0.800757 -0.79486 -0.79486 -0.79486 -0.79486
  spline S2 degree 3 poles (2.9897, 0.42) (3.0543, 0.3464) (3.1943, 0.219) (3.3872, 0.0837) (3.7574, -0.176) (4.273, -0.4422) (4.7124, -0.6375) (5.2684, -0.8846) (5.7621, -1.0583) (6.571, -1.2759) (7.6681, -1.5709) (9.285, -1.9057) (10.7983, -2.1313) (12.3486, -2.3624) (13.7433, -2.4772) (15.0921, -2.5644) (16.7453, -2.6714) (18.3654, -2.7647) (20.5139, -2.8297) (22.493, -2.8895) (24.9582, -2.9109) (27.506, -2.8972) (29.7799, -2.8851) (32.0483, -2.8498) (34.1902, -2.7985) (36.8126, -2.7357) (39.3288, -2.6442) (41.9726, -2.5266) (44.569, -2.411) (47.2437, -2.2742) (49.7746, -2.1475) (52.1544, -2.0283) (54.3796, -1.9201) (56.8136, -1.8047) (59.0608, -1.6981) (61.5509, -1.5807) (64.4566, -1.4428) (69.9758, -1.181) (76.92, -0.8547) (83.3434, -0.5864) (87.9529, -0.3939) (92.2873, -0.2286) (96.4895, -0.064) (101.2103, 0.121) (105.8624, 0.3155) (110.7376, 0.5168) (116.1156, 0.7389) (121.7528, 0.9526) (127.3, 1.1404) (131.5605, 1.2846) (135.7191, 1.4217) (139.6944, 1.5684) (145.3748, 1.778) (150.7153, 2.0131) (156.9225, 2.1285) (160.1948, 2.1893) (163.72, 2.2137) (167.2511, 2.2303) (171.3919, 2.2497) (175.4512, 2.2724) (178.7296, 2.3656) (180.2835, 2.4098) (181.6615, 2.4681) (182.9209, 2.533) knots -0.783322 -0.783322 -0.783322 -0.783322 -0.778142 -0.778142 -0.778142 -0.768195 -0.768195 -0.768195 -0.755608 -0.755608 -0.755608 -0.738537 -0.738537 -0.738537 -0.721048 -0.721048 -0.721048 -0.699613 -0.699613 -0.699613 -0.679868 -0.679868 -0.679868 -0.662246 -0.662246 -0.662246 -0.640672 -0.640672 -0.640672 -0.619485 -0.619485 -0.619485 -0.599563 -0.599563 -0.599563 -0.58117 -0.58117 -0.58117 -0.546233 -0.546233 -0.546233 -0.521162 -0.521162 -0.521162 -0.492997 -0.492997 -0.492997 -0.461927 -0.461927 -0.461927 -0.438064 -0.438064 -0.438064 -0.403967 -0.403967 -0.403967 -0.385991 -0.385991 -0.385991 -0.364912 -0.364912 -0.364912 -0.354921 -0.354921 -0.354921 -0.354921
  spline S3 degree 3 poles (182.9209, 2.533) (181.8753, 2.8143) (180.7522, 3.1063) (179.5028, 3.4129) (176.8181, 4.0717) (173.5306, 4.7965) (170.0047, 5.5188) (166.4626, 6.2444) (162.7518, 6.9595) (159.2882, 7.6111) (155.1437, 8.3909) (151.3487, 9.0818) (147.6957, 9.7206) (143.9527, 10.3752) (140.28, 10.987) (136.4155, 11.5838) (130.3032, 12.5277) (123.7504, 13.4125) (117.3527, 14.1433) (112.3122, 14.7191) (107.4083, 15.2105) (102.6424, 15.6416) (98.0281, 16.059) (93.5117, 16.421) (88.6866, 16.6762) (85.0421, 16.869) (81.1898, 16.9968) (77.299, 17.0516) (73.1641, 17.1099) (69.0475, 17.0885) (65.4867, 17.0124) (63.97, 16.9799) (62.5517, 16.9377) (61.2364, 16.8866) knots -0.236727 -0.236727 -0.236727 -0.236727 -0.22805 -0.22805 -0.22805 -0.209405 -0.209405 -0.209405 -0.190675 -0.190675 -0.190675 -0.168261 -0.168261 -0.168261 -0.145296 -0.145296 -0.145296 -0.108972 -0.108972 -0.108972 -0.080353 -0.080353 -0.080353 -0.052644 -0.052644 -0.052644 -0.031716 -0.031716 -0.031716 -0.009474 -0.009474 -0.009474 0 0 0 0
  spline S4 degree 5 poles (2.9897, 0.42) (3.2959, 0.5113) (3.9165, 0.6914) (4.8716, 0.9537) (6.1935, 1.2878) (7.924, 1.6794) (9.7254, 2.0454) (11.5825, 2.3866) (13.4699, 2.7042) (15.3572, 3.0002) (17.2167, 3.277) (19.0304, 3.5379) (20.7982, 3.7868) (22.5404, 4.0283) (24.2879, 4.2667) (26.0744, 4.5055) (27.9285, 4.7464) (29.8655, 4.9892) (31.8891, 5.2317) (33.9926, 5.471) (36.1602, 5.7042) (38.3678, 5.9288) (40.5851, 6.1431) (42.7814, 6.3464) (44.9313, 6.5384) (47.0192, 6.7191) (49.0456, 6.8882) (51.0316, 7.0456) (53.0081, 7.1908) (55.0055, 7.3235) (57.0448, 7.4437) (59.1255, 7.5512) (61.2209, 7.6466) (63.294, 7.7307) (65.3093, 7.8043) (67.2453, 7.8687) (69.1102, 7.9252) (70.9438, 7.9751) (72.799, 8.0196) (74.7273, 8.0593) (76.7636, 8.0945) (78.909, 8.1243) (81.1396, 8.1472) (83.4178, 8.1619) (85.7031, 8.1668) (87.9623, 8.1611) (90.1818, 8.145) (92.3676, 8.1194) (94.5378, 8.0858) (96.7176, 8.0456) (98.9335, 7.9999) (101.207, 7.9491) (103.5514, 7.8928) (105.9722, 7.8301) (108.4664, 7.76) (111.0226, 7.6819) (113.6208, 7.5955) (116.2315, 7.5015) (118.8198, 7.4014) (121.3514, 7.2969) (123.7982, 7.1898) (126.1443, 7.081) (128.3907, 6.9708) (130.5633, 6.858) (132.7053, 6.7403) (134.8671, 6.615) (137.0959, 6.4797) (139.4265, 6.3328) (141.8693, 6.1742) (144.4088, 6.0051) (147.0128, 5.828) (149.6386, 5.6454) (152.2406, 5.4602) (154.7766, 5.2745) (157.2163, 5.0894) (159.544, 4.9046) (161.7552, 4.7194) (163.8555, 4.5325) (165.8585, 4.3428) (167.7832, 4.1495) (169.653, 3.9526) (171.4925, 3.7529) (173.3255, 3.551) (175.1725, 3.348) (177.0479, 3.1443) (178.9603, 2.9405) (180.5233, 2.7775) (181.7146, 2.6552) (182.5174, 2.5737) (182.9209, 2.533) knots 0 0 0 0 0 0 0.01176471 0.02352941 0.03529412 0.04705882 0.05882353 0.07058824 0.08235294 0.09411765 0.10588235 0.11764706 0.12941176 0.14117647 0.15294118 0.16470588 0.17647059 0.18823529 0.2 0.21176471 0.22352941 0.23529412 0.24705882 0.25882353 0.27058824 0.28235294 0.29411765 0.30588235 0.31764706 0.32941176 0.34117647 0.35294118 0.36470588 0.37647059 0.38823529 0.4 0.41176471 0.42352941 0.43529412 0.44705882 0.45882353 0.47058824 0.48235294 0.49411765 0.50588235 0.51764706 0.52941176 0.54117647 0.55294118 0.56470588 0.57647059 0.58823529 0.6 0.61176471 0.62352941 0.63529412 0.64705882 0.65882353 0.67058824 0.68235294 0.69411765 0.70588235 0.71764706 0.72941176 0.74117647 0.75294118 0.76470588 0.77647059 0.78823529 0.8 0.81176471 0.82352941 0.83529412 0.84705882 0.85882353 0.87058824 0.88235294 0.89411765 0.90588235 0.91764706 0.92941176 0.94117647 0.95294118 0.96470588 0.97647059 0.98823529 1 1 1 1 1 1 construction
  point P0 (10.0423, 2.0974)
  point P1 (18.4182, 3.4489)
  point P2 (25.9781, 4.4911)
  point P3 (35.6221, 5.6443)
  point P4 (46.8596, 6.7039)
  point P5 (56.4979, 7.4092)
  point P6 (66.4709, 7.8422)
  point P7 (74.9764, 8.0623)
  point P8 (86.4632, 8.1634)
  point P9 (98.0008, 8.0186)
  point P10 (111.8166, 7.6545)
  point P11 (126.6735, 7.0541)
  point P12 (138.2667, 6.4053)
  point P13 (153.5666, 5.3624)
  point P14 (165.6182, 4.3633)
  point P15 (174.036, 3.4731)
  point P16 (10.0423, 2.0974)
  point P17 (18.4182, 3.4489)
  point P18 (25.9781, 4.4911)
  point P19 (35.6221, 5.6443)
  point P20 (46.8596, 6.7039)
  point P21 (56.4979, 7.4092)
  point P22 (66.4709, 7.8422)
  point P23 (74.9764, 8.0623)
  point P24 (86.4632, 8.1634)
  point P25 (98.0008, 8.0186)
  point P26 (111.8166, 7.6545)
  point P27 (126.6735, 7.0541)
  point P28 (138.2667, 6.4053)
  point P29 (153.5666, 5.3624)
  point P30 (165.6182, 4.3633)
  point P31 (174.036, 3.4731)
  dimension "d19" = -3
  constraint coincident P16 P0
  constraint coincident P17 P1
  constraint coincident P18 P2
  constraint coincident P19 P3
  constraint coincident P20 P4
  constraint coincident P21 P5
  constraint coincident P22 P6
  constraint coincident P23 P7
  constraint coincident P24 P8
  constraint coincident P25 P9
  constraint coincident P26 P10
  constraint coincident P27 P11
  constraint coincident P28 P12
  constraint coincident P29 P13
  constraint coincident P30 P14
  constraint coincident P31 P15